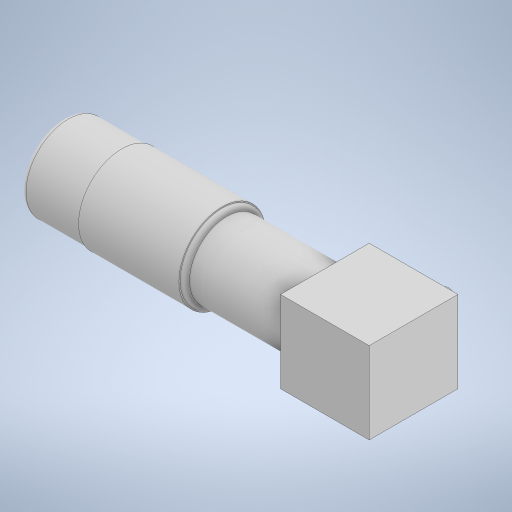
# Autodesk Inventor part: WristMotor
Saved by Autodesk Inventor 2024 (Build 280153000, 153)
## iProperties
Created: 2024-02-01
Part Number: WristMotor
Material: Generic
Document SubType Name: Modeling
Designer: Irwin
Density: 1 g/cm^3
Appearance: Default
Author: Irwin
Autodesk Inventor part; units mm, degrees
ref_plane "YZ Plane" through (0, 0, 0) normal (1, 0, 0) x (0, 1, 0)
ref_plane "XZ Plane" through (0, 0, 0) normal (0, 1, 0) x (-1, 0, 0)
sketch "Sketch1" plane through (0, 0, 0) normal (0, 0, 1) x (1, 0, 0)
  line L0 (-75, 0) -> (75, 0)
  line L1 (-105, 0) -> (105, 0) projected
  point P0 (0, 0)
  dimension "d0" = 150
  dimension "d1" = 75
  constraints: 2 collinear, 2 end point, 1 horizontal
  measures "d0" distance of L0.start L0.end
  measures "d1" distance of L0.end point (0, 0)
ref_plane "Work Plane1" through (75, 0, 0) normal (1, 0, 0) x (0, 1, 0)
sketch "Sketch2" plane through (75, 0, 0) normal (1, 0, 0) x (0, 1, 0)
  line L0 (-17.5, 19) -> (17.5, 19)
  line L1 (17.5, 19) -> (17.5, -19)
  line L2 (17.5, -19) -> (-17.5, -19)
  line L3 (-17.5, -19) -> (-17.5, 19)
  line L4 (-17.5, 19) -> (17.5, -19) construction
  line L5 (17.5, 19) -> (-17.5, -19) construction
  point P0 (0, 0)
  dimension "d2" = 35
  dimension "d3" = 38
  constraints: 12 end point, 2 midpoint, 2 parallel, 1 horizontal, 1 perpendicular
  measures "d2" distance of L1.end L2.end
  measures "d3" distance of L0.end L1.end
extrude "Extrusion1" add sketch "Sketch2" against normal blind 38
sketch "Sketch3" plane through (37, 0, 0) normal (-1, 0, 0) x (0, 0, 1)
  circle A0 centre (0, 0) radius 16
  dimension "d6" = 32
  constraints: 1 centre point, 1 coincident
  measures "d6" diameter of A0
extrude "Extrusion2" add sketch "Sketch3" along normal blind 42
sketch "Sketch4" plane through (-5, 0, 0) normal (-1, 0, 0) x (0, 0, 1)
  circle A0 centre (0, 0) radius 18
  dimension "d9" = 36
  constraints: 1 centre point, 1 coincident
  measures "d9" diameter of A0
extrude "Extrusion3" add sketch "Sketch4" along normal blind 2
sketch "Sketch5" plane through (-7, 0, 0) normal (-1, 0, 0) x (0, 0, 1)
  circle A0 centre (0, 0) radius 18.5
  dimension "d12" = 37
  constraints: 1 centre point, 1 coincident
  measures "d12" diameter of A0
extrude "Extrusion4" add sketch "Sketch5" along normal blind 68
sketch "Sketch6" plane through (-75, 0, 0) normal (-1, 0, 0) x (0, 0, 1)
  circle A0 centre (0, 0) radius 18
  circle A1 centre (0, 0) radius 18.5
  dimension "d15" = 36
  dimension "d16" = 37
  constraints: 2 centre point, 2 coincident
  measures "d15" diameter of A0
  measures "d16" diameter of A1
extrude "Extrusion5" cut sketch "Sketch6" against normal blind 25
fillet "Fillet1" radius 2 2 edges at (-75, 0, -18) (-5, 0, -18)
sketch "Sketch7" plane through (75, -17.5, -19) normal (0, 0, -1) x (-1, 0, 0)
  circle A0 centre (19, 17.5) radius 3
  line L0 (0, 35) -> (38, 35) projected
  line L1 (0, 0) -> (0, 35) projected
  point P0 (75, 17.5)
  dimension "d20" = 6
  dimension "d21" = 17.5
  dimension "d22" = 19
  constraints: 1 centre point
  measures "d20" diameter of A0
  measures "d21" distance from line of L0 A0.centre
  measures "d22" distance from line of L1 A0.centre
extrude "Extrusion6" add sketch "Sketch7" along normal blind 15 separate body
body "Solid1"
body "Solid2"
